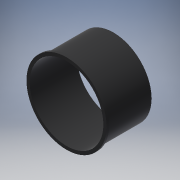
# Autodesk Inventor part: koleso
Saved by Autodesk Inventor 2016 (Build 200138000, 138)
## iProperties
Created: 2015-06-07
Part Number: koleso
Material: ABS Plastic
Document SubType Name: Modeling
Designer: Jufo
Density: 1 g/cm^3
Appearance: Smooth - White
Author: Jufo
Autodesk Inventor part; units mm, degrees
ref_plane "YZ Plane" through (0, 0, 0) normal (1, 0, 0) x (0, 1, 0)
ref_plane "XZ Plane" through (0, 0, 0) normal (0, 1, 0) x (-1, 0, 0)
ref_plane "XY Plane" through (0, 0, 0) normal (0, 0, 1) x (1, 0, 0)
sketch "Sketch4" plane through (0, 0, 0) normal (0, 1, 0) x (-1, 0, 0)
  circle A0 centre (87.8745, -116.8332) radius 29.25
  point P0 (0, 0)
  dimension "d11" = 58.5
  constraints: 1 centre point
  measures "d11" diameter of A0
extrude "Extrusion4" add sketch "Sketch4" along normal blind 36
sketch "Sketch6" plane through (-87.8745, 0, -116.8332) normal (0, -1, 0) x (1, 0, 0)
  circle A0 centre (0, 0) radius 30.75
  point P0 (87.8745, 116.8332)
  dimension "d20" = 61.5
  constraints: 1 centre point
  measures "d20" diameter of A0
extrude "Extrusion6" add sketch "Sketch6" against normal blind 2
sketch "Sketch7" plane through (-87.8745, 36, -116.8332) normal (0, 1, 0) x (1, 0, 0)
  circle A0 centre (0, 0) radius 30.75
  point P0 (87.8745, -116.8332)
  dimension "d23" = 61.5
  constraints: 1 centre point
  measures "d23" diameter of A0
extrude "Extrusion7" add sketch "Sketch7" against normal blind 2
sketch "Sketch5" plane through (-87.8745, 0, -116.8332) normal (0, -1, 0) x (1, 0, 0)
  circle A0 centre (0, 0) radius 28
  circle A1 centre (0, 0) radius 29.25 projected
  point P0 (87.8745, 116.8332)
  dimension "d16" = 0
  dimension "d17" = 0
  dimension "d26" = 56
  constraints: 1 centre point
  measures "d16" distance of A1.centre A0.centre
  measures "d17" distance of A1.centre A0.centre
  measures "d26" diameter of A0
extrude "Extrusion5" cut sketch "Sketch5" against normal blind 36 contours A0
sketch "Sketch8" plane through (-87.8745, 0, -116.8332) normal (0, -1, 0) x (1, 0, 0)
  circle A0 centre (0, 0) radius 8.5
  circle A1 centre (0, 0) radius 28 projected
  line L0 (28, 0) -> (28, 2.25)
  line L1 (28, 0) -> (28, -2.25)
  line L2 (8.5, 0) -> (8.5, 4.3)
  line L3 (8.5, 0) -> (8.5, -4.3)
  line L4 (8.5, 4.3) -> (28, 2.25)
  line L5 (8.5, -4.3) -> (28, -2.25)
  arc A2 (27.9087, -2.2596) -> (27.9087, 2.2596) centre (0, 0) ccw
  line L6 (-1.4629, 9.4128) -> (6.5126, 27.3249)
  line L7 (2.6266, 8.084) -> (-1.4629, 9.4128)
  line L8 (2.6266, 8.084) -> (6.7162, 6.7552)
  line L9 (6.7162, 6.7552) -> (10.7924, 25.9343)
  arc A3 (10.7733, 25.8445) -> (6.4752, 27.241) centre (0, 0) ccw
  line L10 (-9.4041, 1.5174) -> (-23.975, 14.6377)
  line L11 (-6.8766, 4.9962) -> (-9.4041, 1.5174)
  line L12 (-6.8766, 4.9962) -> (-4.3492, 8.4749)
  line L13 (-4.3492, 8.4749) -> (-21.33, 18.2783)
  arc A4 (-21.2504, 18.2324) -> (-23.9068, 14.5763) centre (0, 0) ccw
  line L14 (-4.3492, -8.4749) -> (-21.33, -18.2783)
  line L15 (-6.8766, -4.9962) -> (-4.3492, -8.4749)
  line L16 (-6.8766, -4.9962) -> (-9.4041, -1.5174)
  line L17 (-9.4041, -1.5174) -> (-23.975, -14.6377)
  arc A5 (-23.9068, -14.5763) -> (-21.2504, -18.2324) centre (0, 0) ccw
  line L18 (6.7162, -6.7552) -> (10.7924, -25.9343)
  line L19 (2.6266, -8.084) -> (6.7162, -6.7552)
  line L20 (2.6266, -8.084) -> (-1.4629, -9.4128)
  line L21 (-1.4629, -9.4128) -> (6.5126, -27.3249)
  arc A6 (6.4752, -27.241) -> (10.7733, -25.8445) centre (0, 0) ccw
  line L22 (-1.4629, 9.4128) -> (-4.3492, 8.4749)
  line L23 (-9.4041, 1.5174) -> (-9.4041, -1.5174)
  line L24 (-4.3492, -8.4749) -> (-1.4629, -9.4128)
  line L25 (6.7162, -6.7552) -> (8.5, -4.3)
  line L26 (8.5, 4.3) -> (6.7162, 6.7552)
  line L27 (6.7162, 6.7552) -> (-1.4629, 9.4128)
  line L28 (-4.3492, 8.4749) -> (-9.4041, 1.5174)
  line L29 (-9.4041, -1.5174) -> (-4.3492, -8.4749)
  line L30 (-1.4629, -9.4128) -> (6.7162, -6.7552)
  line L31 (8.5, -4.3) -> (8.5, 4.3)
  point P0 (87.8745, 116.8332)
  point P1 (8.6525, 26.6296)
  point P2 (-22.6525, 16.458)
  point P3 (-22.6525, -16.458)
  point P4 (8.6525, -26.6296)
  dimension "d27" = 17
  dimension "d29" = 2.25
  dimension "d30" = 2.25
  dimension "d31" = 4.3
  dimension "d32" = 4.3
  dimension "d35" = 360
  constraints: 64 end point, 18 point on circle, 10 point on line, 6 vertical, 5 centre point, 3 collinear, 2 tangent, 1 horizontal alignment, 73 other
  measures "d29" distance of L0.start L0.end
  measures "d30" distance of L0.start L1.end
  measures "d31" distance of L2.start L2.end
  measures "d32" distance of L2.start L3.end
extrude "Extrusion8" add sketch "Sketch8" against normal blind 8 contours A0 | L3 L25 L19 A0 | A0 L8 L26 L2 | L2 L4 A1 L5 L3 | A0 L12 L22 L7 | L7 L6 A1 L9 L8 | L20 L24 L15 A0 | L19 L18 A1 L21 L20 | A0 L16 L23 L11 | L11 L10 A1 L13 L12 | L15 L14 A1 L17 L16
sketch "Sketch9" plane through (-87.8745, 0, -116.8332) normal (0, -1, 0) x (1, 0, 0)
  circle A0 centre (0, 0) radius 6.25
  point P0 (87.8745, 116.8332)
  dimension "d39" = 12.5
  constraints: 1 centre point
  measures "d39" diameter of A0
extrude "Extrusion9" cut sketch "Sketch9" against normal blind 2.5
fillet "Fillet1" radius 3 1 edges at (-94.1245, 0, -116.8332)
sketch "Sketch10" plane through (-87.8745, 2.5, -116.8332) normal (0, -1, 0) x (1, 0, 0)
  circle A0 centre (0, 0) radius 2
  point P0 (87.8745, 116.8332)
  dimension "d43" = 4
  constraints: 1 centre point
  measures "d43" diameter of A0
extrude "Extrusion10" cut sketch "Sketch10" against normal blind 50
sketch "Sketch11" plane through (-87.8745, 8, -116.8332) normal (0, 1, 0) x (1, 0, 0)
  circle A0 centre (0, 0) radius 9.208
  circle A1 centre (0, 0) radius 2 projected
  circle A2 centre (0, 0) radius 7.208
  circle A3 centre (0, 0) radius 9.208 projected
  line L0 (0, 7.208) -> (6.2423, 3.604)
  line L1 (6.2423, 3.604) -> (6.2423, -3.604)
  line L2 (6.2423, -3.604) -> (0, -7.208)
  line L3 (0, -7.208) -> (-6.2423, -3.604)
  line L4 (-6.2423, -3.604) -> (-6.2423, 3.604)
  line L5 (-6.2423, 3.604) -> (0, 7.208)
  point P0 (87.8745, -116.8332)
  dimension "d46" = 2
  dimension "d47" = 0
  dimension "d48" = 0
  dimension "d49" = 0
  constraints: 12 end point, 2 coincident, 1 centre point, 1 vertical alignment, 15 other
  measures "d47" radial gap between concentric circles of A3 A0
  measures "d48" distance of point (0, 0) A0.centre
  measures "d49" distance of A0.centre point (0, 0)
extrude "Extrusion11" add sketch "Sketch11" along normal blind 5 contours A0 | A2 L1 | L0 A2 | A2 L2 | L5 A2 | A2 L3 | L4 A2
equation "\"d30\" = d29"
equation "\"d32\" = d31"
body "Solid2"
